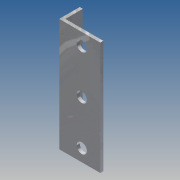
# Autodesk Inventor part: Z-Stage_Wheel_plate
Saved by Autodesk Inventor 2015 SP1 (Build 190203100, 203)
## iProperties
Created: 2015-03-05
Part Number: Z-Stage_Wheel_plate
Material: Aluminium 6061
Document SubType Name: Modeling
Designer: Marc
Mass: 5.77125 g
Surface Area: 30.855 cm^2
Volume: 2.1375 cm^3
Density: 2.7 g/cm^3
Appearance: Aluminium - flach
Author: Marc
Autodesk Inventor part; units mm, degrees
ref_plane "YZ Plane" through (0, 0, 0) normal (1, 0, 0) x (0, 1, 0)
ref_plane "XZ Plane" through (0, 0, 0) normal (0, 1, 0) x (-1, 0, 0)
ref_plane "XY Plane" through (0, 0, 0) normal (0, 0, 1) x (1, 0, 0)
sketch "Skizze1" plane through (0, 0, 0) normal (0, 0, 1) x (1, 0, 0)
  line L0 (-14, 0) -> (14, 0) projected
  line L1 (0, -2.75) -> (0, 11.25) projected
  line L2 (-10, -0.75) -> (10, -0.75)
  line L3 (10, -0.75) -> (10, 0.75)
  line L4 (10, 0.75) -> (-10, 0.75)
  line L5 (-10, 0.75) -> (-10, -0.75)
  line L6 (-10, -0.75) -> (-8.5, -0.75)
  line L7 (-8.5, -0.75) -> (-8.5, 9.25)
  line L8 (-8.5, 9.25) -> (-10, 9.25)
  line L9 (-10, 9.25) -> (-10, -0.75)
  point P0 (0, 0)
  dimension "d0" = 20
  dimension "d1" = 1.5
  dimension "d2" = 1.5
  dimension "d3" = 10
  constraints: 16 end point, 4 parallel, 2 horizontal, 2 perpendicular, 2 other
  measures "d0" distance of L4.end L3.end
  measures "d1" distance of L3.end L2.end
  measures "d2" distance of L8.end L7.end
  measures "d3" distance of L7.end L6.end
extrude "Extrusion1" add sketch "Skizze1" along normal blind 55
sketch "Skizze2" plane through (-8.5, 0.75, 0) normal (0, 1, 0) x (1, 0, 0)
  line L0 (0, -55) -> (0, 0) projected
  line L1 (18.5, -55) -> (0, -55) projected
  line L2 (18.5, 0) -> (18.5, -55) projected
  line L3 (18.5, 0) -> (0, 0) projected
  circle A0 centre (9.5, -49) radius 2.5
  circle A1 centre (9.5, -6) radius 2.5
  circle A2 centre (9.5, -27.5) radius 2.5
  line L4 (18.5, -55) -> (0, -55) projected
  line L5 (18.5, 0) -> (0, 0) projected
  point P0 (8.5, 0)
  dimension "d6" = 5
  dimension "d7" = 5
  dimension "d8" = 6
  dimension "d9" = 6
  dimension "d10" = 9
  dimension "d13" = 5
  dimension "d15" = 55
  dimension "d16" = 27.5
  constraints: 3 centre point, 2 vertical alignment
  measures "d6" diameter of A0
  measures "d7" diameter of A1
  measures "d8" distance from line of L1 A0.centre
  measures "d9" distance from line of L3 A1.centre
  measures "d10" distance from line of L2 A0.centre
  measures "d13" diameter of A2
  measures "d15" distance of L0.start L0.end
  measures "d16" distance from line of L3 A2.centre
extrude "Extrusion2" cut sketch "Skizze2" against normal blind 1.5 contours A0 | A1 | A2
equation "\"d9\" = d8"
equation "\"d16\" = 0.5 * d15"
